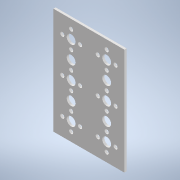
# Autodesk Inventor part: Part4
Saved by Autodesk Inventor 2020.1 (Build 241239000, 239)
## iProperties
Created: 2019-12-06
Part Number: Part4
Material: Generic
Document SubType Name: Modeling
Designer: tbloo
Density: 1 g/cm^3
Appearance: Default
Author: tbloo
Autodesk Inventor part; units mm, degrees
ref_plane "YZ Plane" through (0, 0, 0) normal (1, 0, 0) x (0, 1, 0)
ref_plane "XZ Plane" through (0, 0, 0) normal (0, 1, 0) x (-1, 0, 0)
ref_plane "XY Plane" through (0, 0, 0) normal (0, 0, 1) x (1, 0, 0)
sketch "Sketch1" plane through (0, 0, 0) normal (0, 0, 1) x (1, 0, 0)
  line L0 (32, 0) -> (32, -96) projected
  line L1 (-32, 0) -> (-32, -96) projected
  line L2 (32, 0) -> (-32, 0)
  line L3 (-32, 0) -> (-32, -96)
  line L4 (-32, -96) -> (32, -96)
  line L5 (32, -96) -> (32, 0)
  circle A0 centre (24, -16) radius 1.85 projected
  circle A1 centre (16, -8) radius 1.85 projected
  circle A2 centre (16, -16) radius 4 projected
  circle A3 centre (16, -24) radius 1.85 projected
  circle A4 centre (8, -16) radius 1.85 projected
  circle A5 centre (16, -32) radius 4 projected
  circle A6 centre (16, -40) radius 1.85 projected
  circle A7 centre (16, -48) radius 4 projected
  circle A8 centre (24, -48) radius 1.85 projected
  circle A9 centre (16, -56) radius 1.85 projected
  circle A10 centre (8, -48) radius 1.85 projected
  circle A11 centre (16, -64) radius 4 projected
  circle A12 centre (16, -72) radius 1.85 projected
  circle A13 centre (24, -80) radius 1.85 projected
  circle A14 centre (16, -88) radius 1.85 projected
  circle A15 centre (8, -80) radius 1.85 projected
  circle A16 centre (16, -80) radius 4 projected
  circle A17 centre (-8, -80) radius 1.85 projected
  circle A18 centre (-16, -80) radius 4 projected
  circle A19 centre (-16, -72) radius 1.85 projected
  circle A20 centre (-16, -88) radius 1.85 projected
  circle A21 centre (-24, -80) radius 1.85 projected
  circle A22 centre (-16, -64) radius 4 projected
  circle A23 centre (-16, -56) radius 1.85 projected
  circle A24 centre (-8, -48) radius 1.85 projected
  circle A25 centre (-16, -40) radius 1.85 projected
  circle A26 centre (-24, -48) radius 1.85 projected
  circle A27 centre (-16, -48) radius 4 projected
  circle A28 centre (-16, -32) radius 4 projected
  circle A29 centre (-16, -24) radius 1.85 projected
  circle A30 centre (-8, -16) radius 1.85 projected
  circle A31 centre (-16, -8) radius 1.85 projected
  circle A32 centre (-24, -16) radius 1.85 projected
  circle A33 centre (-16, -16) radius 4 projected
  point P0 (0, 0)
  constraints: 8 end point, 2 parallel, 1 horizontal, 1 perpendicular
extrude "Extrusion1" add sketch "Sketch1" along normal blind 2
sketch "Sketch2" plane through (0, 0, 2) normal (0, 0, 1) x (1, 0, 0)
  circle A0 centre (24, -32) radius 1.85 projected
  circle A1 centre (8, -32) radius 1.85 projected
  circle A2 centre (8, -64) radius 1.85 projected
  circle A3 centre (24, -64) radius 1.85 projected
  circle A4 centre (-8, -32) radius 1.85 projected
  circle A5 centre (-24, -32) radius 1.85 projected
  circle A6 centre (-8, -64) radius 1.85 projected
  circle A7 centre (-24, -64) radius 1.85 projected
  point P0 (0, 0)
extrude "Extrusion2" cut sketch "Sketch2" against normal through all
sketch "Sketch3" plane through (0, 0, 2) normal (0, 0, 1) x (1, 0, 0)
  circle A0 centre (0, -8) radius 1.85 projected
  circle A1 centre (0, -24) radius 1.85 projected
  circle A2 centre (0, -32) radius 4 projected
  circle A3 centre (0, -40) radius 1.85 projected
  circle A4 centre (0, -16) radius 4 projected
  circle A5 centre (0, -48) radius 4 projected
  circle A6 centre (0, -56) radius 1.85 projected
  circle A7 centre (0, -64) radius 4 projected
  circle A8 centre (0, -72) radius 1.85 projected
  circle A9 centre (0, -80) radius 4 projected
  circle A10 centre (0, -88) radius 1.85 projected
  point P0 (0, 0)
extrude "Extrusion3" cut sketch "Sketch3" against normal through all
body "Solid1"
